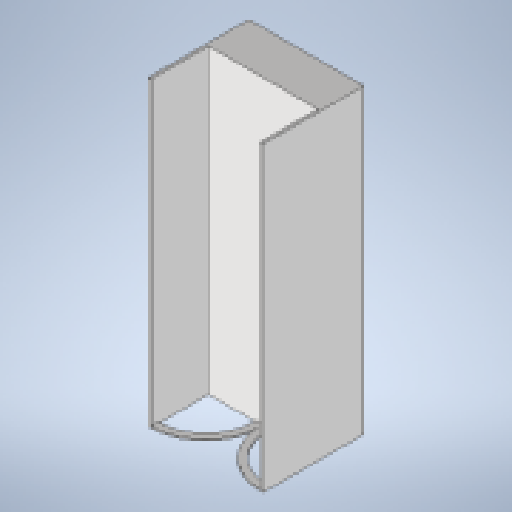
# Autodesk Inventor part: Electrical box 4
Saved by Autodesk Inventor 2025.4 (Build 294407000, 407)
## iProperties
Created: 2026-01-26
Part Number: Electrical box 4
Material: Generic
Document SubType Name: Modeling
Designer: admin
Density: 1 g/cm^3
Appearance: Default
Author: admin
Autodesk Inventor part; units mm, degrees
ref_plane "YZ Plane" through (0, 0, 0) normal (1, 0, 0) x (0, 1, 0)
ref_plane "XZ Plane" through (0, 0, 0) normal (0, 1, 0) x (-1, 0, 0)
ref_plane "XY Plane" through (0, 0, 0) normal (0, 0, 1) x (1, 0, 0)
sketch "Sketch1" plane through (0, 0, 0) normal (0, 1, 0) x (-1, 0, 0)
  line L0 (0, 0) -> (-400, 0)
  line L1 (-400, 0) -> (-400, 300)
  line L2 (-400, 300) -> (0, 300)
  line L3 (0, 300) -> (0, 0)
  line L4 (0, 300) -> (-20, 300)
  line L5 (-400, 300) -> (-380, 300)
  line L6 (-380, 300) -> (-380, 700)
  line L7 (-380, 700) -> (-400, 700)
  line L8 (-400, 700) -> (-400, 300)
  point P0 (-380, 300)
  dimension "d0" = 400
  dimension "d1" = 300
  dimension "d9" = 400
  dimension "d10" = 20
  constraints: 18 end point, 4 parallel, 3 horizontal, 2 perpendicular
  measures "d0" distance of L0.start L0.end
  measures "d1" distance of L2.end L0.start
  measures "d9" distance of L7.end L1.end
  measures "d10" distance of L6.end L7.end
extrude "Extrusion1" add sketch "Sketch1" along normal blind 2100
sketch "Sketch3" plane through (0, 0, 0) normal (0, 1, 0) x (-1, 0, 0)
  line L0 (0, 300) -> (-380, 300) projected
  line L1 (-380, 300) -> (-380, 700) projected
  line L2 (-380, 700) -> (-400, 700) projected
  line L3 (-400, 700) -> (-400, 0) projected
  line L4 (-400, 0) -> (0, 0) projected
  line L5 (0, 0) -> (0, 300) projected
  arc A0 (0, 300) -> (-380, 700) centre (-380, 319.5) ccw
  arc A1 (-50.0758, 300) -> (-380, 650) centre (-380, 319.5) ccw
  dimension "d11" = 50
  constraints: 4 point on circle, 3 point on line, 2 centre point
  measures "d11" radial gap between concentric circles of A0 A1
extrude "Extrusion3" add sketch "Sketch3" along normal blind 10 contours L0 A1 L1 A0
mirror "Mirror1" about plane through (0, 0, 0) normal (-1, 0, 0) of "Extrusion1", "Extrusion3"
equation "\"d9\" = d0"
body "Solid1"
